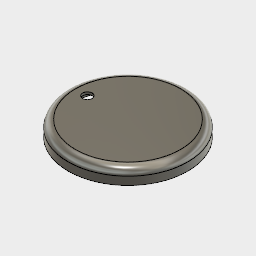
03 Desk Lamp v3 (Autodesk Fusion 360 design; units mm, degrees)
Autodesk Fusion 360 part; units mm, degrees
sketch "LampBase" plane through (0, 0, 0) normal (0, 0, 1) x (1, 0, 0)
  line L0 (0, 0) -> (125, 0)
  line L1 (125, 0) -> (125, 32)
  line L2 (125, 32) -> (0, 32)
  line L3 (0, 32) -> (0, 0)
  dimension "d1" = 125
  dimension "d2" = 32
  measures "d1" distance of L0.start L0.end
  measures "d2" distance of L0.start L2.end
revolve "Revolve1" add sketch "LampBase" angle 360 about axis through (0, 32, 0) along (0, -1, 0)
fillet "Fillet1" radius 15 1 edges at (-116.5409, 32, -45.2019)
shell "Shell1" thickness 5 removed faces 1 at (-15.2225, 0, 33.3824)
sketch "Sketch2" plane through (0, 32, 0) normal (0, 1, 0) x (-1, 0, 0)
  circle A0 centre (0, 0) radius 110
  circle A1 centre (85, 0) radius 10
  dimension "d6" = 20
  dimension "d7" = 85
  measures "d6" diameter of A1
  measures "d7" distance of A0.centre A1.centre
extrude "Extrude1" cut sketch "Sketch2" against normal blind 10 contours A1
